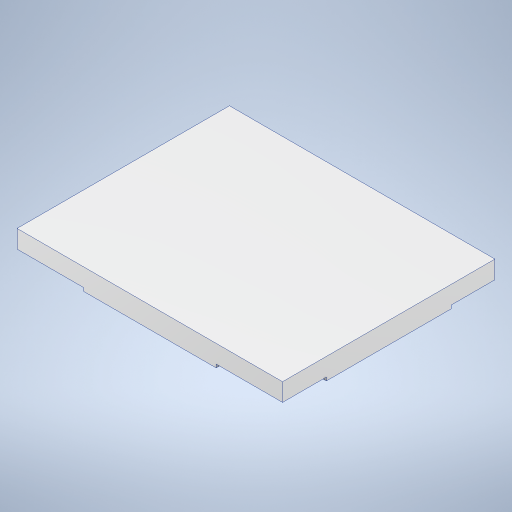
# Autodesk Inventor part: Y_karetka
Saved by Autodesk Inventor 2024 (Build 280153000, 153)
## iProperties
Created: 2023-08-21
Part Number: Y_karetka
Material: Aluminum 6061
Document SubType Name: Modeling
Designer: KirikDK
Mass: 1529.39 g
Surface Area: 1104.64 cm^2
Volume: 566.44 cm^3
Density: 2.7 g/cm^3
Appearance: Aluminum - Flat
Author: KirikDK
Autodesk Inventor part; units mm, degrees
ref_plane "YZ Plane" through (0, 0, 0) normal (1, 0, 0) x (0, 1, 0)
ref_plane "XZ Plane" through (0, 0, 0) normal (0, 1, 0) x (-1, 0, 0)
ref_plane "XY Plane" through (0, 0, 0) normal (0, 0, 1) x (1, 0, 0)
sketch "Sketch1" plane through (0, 0, 0) normal (0, 1, 0) x (-1, 0, 0)
  line L0 (13.84, 90.8) -> (-186.16, 90.8)
  line L1 (-186.16, 90.8) -> (-186.16, -69.2)
  line L2 (-186.16, -69.2) -> (13.84, -69.2)
  line L3 (13.84, -69.2) -> (13.84, 90.8)
  point P0 (0, 0)
  dimension "d0" = 160
  dimension "d1" = 200
  constraints: 8 end point, 2 parallel, 1 horizontal, 1 perpendicular
  measures "d0" distance of L2.end L0.start
  measures "d1" distance of L1.end L2.end
extrude "Extrusion1" add sketch "Sketch1" along normal blind 11
sketch "Sketch2" plane through (186.16, 0, 90.8) normal (1, 0, 0) x (0, 0, -1)
  line L0 (0, 0) -> (0, 11) projected
  line L1 (0, 0) -> (-12, 0)
  line L2 (-12, 0) -> (-12, 60)
  line L3 (-12, 60) -> (0, 60)
  line L4 (0, 60) -> (0, 0)
  line L5 (160, 0) -> (160, 11) projected
  line L6 (160, 0) -> (172, 0)
  line L7 (172, 0) -> (172, 60)
  line L8 (172, 60) -> (160, 60)
  line L9 (160, 60) -> (160, 0)
  point P0 (90.8, 0)
  point P1 (0, 11)
  dimension "d4" = 60
  dimension "d5" = 60
  dimension "d6" = 12
  dimension "d17" = 12
  constraints: 16 end point, 5 equal length, 2 horizontal, 2 perpendicular, 1 collinear
  measures "d4" distance between parallel lines of L1 L3
  measures "d5" distance between parallel lines of L6 L8
  measures "d6" distance of L2.end L3.end
  measures "d17" distance of L7.end L8.end
extrude "Extrusion2" add sketch "Sketch2" against normal up to surface (200 mm away)
sketch "Sketch3" plane through (0, 0, 0) normal (0, -1, 0) x (1, 0, 0)
  line L0 (186.16, 102.8) -> (186.16, -81.2) projected
  line L1 (186.16, 102.8) -> (-13.84, 102.8) projected
  line L2 (-13.84, -81.2) -> (-13.84, 102.8) projected
  line L3 (186.16, -81.2) -> (-13.84, -81.2) projected
  point P0 (0, 0)
extrude "Extrusion3" add sketch "Sketch3" along normal blind 5
sketch "Sketch7" plane through (0, 11, 0) normal (0, 1, 0) x (1, 0, 0)
  line L0 (186.16, -90.8) -> (-13.84, -90.8) projected
  line L1 (36.16, -90.8) -> (136.16, -90.8)
  line L2 (136.16, -90.8) -> (136.16, -65.8)
  line L3 (136.16, -65.8) -> (36.16, -65.8)
  line L4 (36.16, -65.8) -> (36.16, -90.8)
  line L5 (186.16, 69.2) -> (-13.84, 69.2) projected
  line L6 (36.16, 69.2) -> (136.16, 69.2)
  line L7 (136.16, 69.2) -> (136.16, 44.2)
  line L8 (136.16, 44.2) -> (36.16, 44.2)
  line L9 (36.16, 44.2) -> (36.16, 69.2)
  line L10 (-13.84, 69.2) -> (-13.84, -90.8) projected
  line L11 (186.16, -90.8) -> (186.16, 69.2) projected
  point P0 (0, 0)
  point P1 (136.16, 56.7)
  dimension "d18" = 25
  dimension "d19" = 25
  dimension "d20" = 50
  dimension "d21" = 50
  dimension "d22" = 50
  dimension "d23" = 50
  constraints: 16 end point, 4 parallel, 2 horizontal, 2 perpendicular, 2 point on line, 1 midpoint
  measures "d18" distance between parallel lines of L0 L3
  measures "d19" distance between parallel lines of L5 L8
  measures "d20" distance between parallel lines of L10 L9
  measures "d21" distance from line of L11 point (136.16, 56.7)
  measures "d22" distance between parallel lines of L10 L4
  measures "d23" distance between parallel lines of L11 L2
extrude "Extrusion6" add sketch "Sketch7" along normal blind 10 contours L0 L4 L3 L2 | L7 L8 L9 L5
fillet "Fillet1" radius 4 4 edges at (36.16, 16, -69.2) (36.16, 16, 90.8) (136.16, 16, -69.2) (136.16, 16, 90.8)
fillet "Fillet2" radius 10 4 edges at (138.16, 21, -69.2) (34.16, 21, -69.2) (34.16, 21, 90.8) (138.16, 21, 90.8)
sketch "Sketch8" plane through (-13.84, 11, 90.8) normal (-1, 0, 0) x (0, 0, 1)
  line L0 (-160, 0) -> (0, 0)
  line L1 (0, 0) -> (0, -19)
  line L2 (0, -19) -> (-160, -19)
  line L3 (-160, -19) -> (-160, 0)
  line L4 (-172, 49) -> (12, 49)
  line L5 (12, 49) -> (12, -16)
  line L6 (12, -16) -> (-172, -16)
  line L7 (-172, -16) -> (-172, 49)
  point P0 (-90.8, -11)
  point P1 (0, -16)
  point P2 (-160, -16)
  constraints: 16 end point, 4 parallel, 2 horizontal, 2 perpendicular
extrude "Extrusion7" cut sketch "Sketch8" against normal blind 1000 contours L3 L6 L7 L4 L5 L1 L0
sketch "Sketch10" plane through (0, -5, 0) normal (0, -1, 0) x (1, 0, 0)
  line L0 (186.16, -69.2) -> (-13.84, -69.2) projected
  line L1 (-13.84, -69.2) -> (36.16, -69.2)
  line L2 (36.16, -69.2) -> (36.16, -36.2)
  line L3 (36.16, -36.2) -> (-13.84, -36.2)
  line L4 (-13.84, -36.2) -> (-13.84, -69.2)
  line L5 (186.16, -69.2) -> (136.16, -69.2)
  line L6 (136.16, -69.2) -> (136.16, -36.2)
  line L7 (136.16, -36.2) -> (186.16, -36.2)
  line L8 (186.16, -36.2) -> (186.16, -69.2)
  line L9 (186.16, 90.8) -> (136.16, 90.8)
  line L10 (136.16, 90.8) -> (136.16, 57.8)
  line L11 (136.16, 57.8) -> (186.16, 57.8)
  line L12 (186.16, 57.8) -> (186.16, 90.8)
  line L13 (-13.84, 90.8) -> (36.16, 90.8)
  line L14 (36.16, 90.8) -> (36.16, 57.8)
  line L15 (36.16, 57.8) -> (-13.84, 57.8)
  line L16 (-13.84, 57.8) -> (-13.84, 90.8)
  line L17 (186.16, 90.8) -> (-13.84, 90.8) projected
  point P0 (0, 0)
  dimension "d30" = 50
  dimension "d31" = 50
  dimension "d32" = 50
  dimension "d33" = 50
  dimension "d34" = 33
  dimension "d35" = 33
  dimension "d36" = 0
  constraints: 32 end point, 10 parallel, 4 horizontal, 4 perpendicular, 4 point on line
  measures "d30" distance of L6.end L7.end
  measures "d31" distance of L10.end L11.end
  measures "d32" distance of L14.end L15.end
  measures "d33" distance of L2.end L3.end
  measures "d34" distance of L5.end L6.end
  measures "d35" distance of L9.end L10.end
  measures "d36" distance between parallel lines of L17 L9
extrude "Extrusion8" cut sketch "Sketch10" against normal blind 2.5
body "Solid1"
